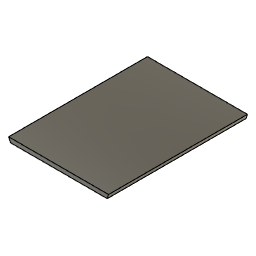
top v3 (Autodesk Fusion 360 design; units mm, degrees)
Autodesk Fusion 360 part; units mm, degrees
sketch "Esquisse1" plane through (0, 0, 0) normal (0, 1, 0) x (1, 0, 0)
  line L0 (2.0601, 0) -> (93.7885, 0)
  line L1 (95, -4) -> (0, -4)
  line L2 (0, -4) -> (2.0601, 0)
  line L3 (95, -4) -> (93.7885, 0)
  dimension "d3" = 62.75
  dimension "d4" = 73.15
  constraint horizontal L0
  measures "d3" angle of L1 L2
  measures "d4" angle of L1 L3
extrude "Extrusion1" add sketch "Esquisse1" along normal blind 132
